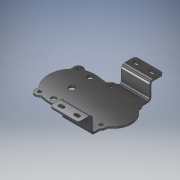
# Autodesk Inventor part: STEEL SIDE REDUCTION FRONT PLATE
Saved by Autodesk Inventor 2017 (Build 210142000, 142)
## iProperties
Part Number: STEEL SIDE REDUCTION FRONT PLATE
Material: Genérico
Document SubType Name: Modeling
Designer: Cristian
Density: 1 g/cm^3
Appearance: Valor por defecto
Author: Cristian
Autodesk Inventor part; units mm, degrees
ref_plane "XZ Plane" through (0, 0, 0) normal (0, 1, 0) x (-1, 0, 0)
ref_plane "XY Plane" through (0, 0, 0) normal (0, 0, 1) x (1, 0, 0)
sketch "Boceto1" plane through (0, 0, 0) normal (0, 0, 1) x (1, 0, 0)
  circle A0 centre (0, 0) radius 57.15
  circle A1 centre (101.6, 0) radius 44.45
  circle A2 centre (-31.75, 47.519) radius 11.1125
  circle A3 centre (-31.75, -47.519) radius 11.1125
  circle A4 centre (114.3, 42.5971) radius 11.1125
  circle A5 centre (114.3, -42.5971) radius 11.1125
  line L0 (7.1437, 56.7018) -> (107.1562, 44.1014)
  circle A6 centre (44.45, 52.0016) radius 11.1125
  line L1 (7.1437, -56.7018) -> (107.1562, -44.1014)
  circle A7 centre (44.45, -52.0016) radius 11.1125
  dimension "d0" = 114.3
  dimension "d1" = 88.9
  dimension "d2" = 203.2
  dimension "d3" = 22.225
  dimension "d4" = 22.225
  dimension "d7" = 22.225
  dimension "d8" = 22.225
  dimension "d11" = 22.225
  dimension "d13" = 0
  dimension "d14" = 22.225
  dimension "d35" = 31.75
  dimension "d36" = 31.75
  dimension "d37" = 44.45
  dimension "d38" = 44.45
  dimension "d39" = 12.7
  dimension "d40" = 12.7
  constraints: 8 centre point, 8 point on circle, 4 end point, 4 tangent, 2 point on line, 1 coincident
  measures "d0" diameter of A0
  measures "d1" diameter of A1
  measures "d3" diameter of A2
  measures "d4" diameter of A3
  measures "d7" diameter of A4
  measures "d8" diameter of A5
  measures "d11" diameter of A6
  measures "d13" vertical distance of point (0, 0) A1.centre
  measures "d14" diameter of A7
  measures "d35" horizontal distance of A0.centre A3.centre
  measures "d36" horizontal distance of A0.centre A2.centre
  measures "d37" horizontal distance of point (0, 0) A7.centre
  measures "d38" horizontal distance of point (0, 0) A6.centre
  measures "d39" horizontal distance of A1.centre A5.centre
  measures "d40" horizontal distance of A1.centre A4.centre
extrude "Extrusión1" add sketch "Boceto1" along normal blind 4.445
ref_plane "Plano de trabajo1" through (50.8, 0, 0) normal (1, 0, 0) x (0, 1, 0)
sketch "Boceto3" plane through (50.8, 0, 0) normal (1, 0, 0) x (0, 1, 0)
  line L0 (0, 0) -> (0, 4.445)
  line L1 (-52.7651, 4.445) -> (-56.7018, 4.445) projected
  line L2 (0, 4.445) -> (69.85, 4.445)
  line L3 (69.85, 4.445) -> (69.85, 44.45)
  line L4 (69.85, 44.45) -> (104.775, 44.45)
  line L5 (104.775, 44.45) -> (104.775, 40.005)
  line L6 (104.775, 40.005) -> (74.295, 40.005)
  line L7 (74.295, 40.005) -> (74.295, 0)
  line L8 (74.295, 0) -> (0, 0)
  point P0 (37.2916, 4.445)
  point P1 (-37.2916, 4.445)
  dimension "d28" = 4.445
  dimension "d29" = 4.445
  dimension "d30" = 69.85
  dimension "d31" = 44.45
  dimension "d32" = 104.775
  constraints: 16 end point, 6 perpendicular, 1 horizontal, 1 point on line
  measures "d28" distance between parallel lines of L7 L3
  measures "d29" distance between parallel lines of L4 L6
  measures "d30" distance of L0.end L2.end
  measures "d31" distance between parallel lines of L4 L8
  measures "d32" distance between parallel lines of L0 L5
extrude "Extrusión3" add sketch "Boceto3" along normal blind 69.85
fillet "Empalme3" radius 4.445 2 edges at (85.725, 69.85, 4.445) (85.725, 74.295, 40.005)
fillet "Empalme4" radius 8.89 2 edges at (85.725, 69.85, 44.45) (85.725, 74.295, 0)
sketch "Boceto4" plane through (50.8, 104.775, 44.45) normal (0, 0, 1) x (1, 0, 0)
  circle A0 centre (12.7254, -12.7254) radius 4.191
  circle A1 centre (19.0246, -12.7254) radius 4.191
  circle A2 centre (57.1246, -12.7254) radius 4.191
  circle A3 centre (50.8254, -12.7254) radius 4.191
  line L0 (57.1246, -8.5344) -> (50.8254, -8.5344)
  line L1 (57.1246, -16.9164) -> (50.8254, -16.9164)
  line L2 (0, 0) -> (69.85, 0) projected
  line L3 (69.85, 0) -> (69.85, -26.035) projected
  line L4 (19.0246, -8.5344) -> (12.7254, -8.5344)
  line L5 (12.7254, -16.9164) -> (19.0246, -16.9164)
  line L6 (0, -26.035) -> (0, 0) projected
  point P0 (-50.8, -104.775)
  point P1 (6.35, 0)
  point P2 (63.5, 0)
  point P3 (69.85, -6.35)
  point P4 (0, -6.35)
  dimension "d44" = 8.382
  dimension "d45" = 8.382
  dimension "d46" = 14.6812
  dimension "d47" = 8.5344
  dimension "d48" = 12.7254
  dimension "d49" = 8.382
  dimension "d50" = 8.382
  dimension "d51" = 14.6812
  dimension "d52" = 8.5344
  dimension "d53" = 12.7254
  constraints: 8 end point, 8 point on circle, 7 tangent, 4 centre point, 1 parallel
  measures "d44" diameter of A2
  measures "d45" diameter of A3
  measures "d47" distance between parallel lines of L2 L0
  measures "d48" distance from line of L3 A2.centre
  measures "d49" diameter of A1
  measures "d50" diameter of A0
  measures "d52" distance between parallel lines of L2 L4
  measures "d53" distance from line of L6 A0.centre
extrude "Extrusión4" cut sketch "Boceto4" against normal up to surface (4.445 mm away)
fillet "Empalme5" radius 6.35 2 edges at (120.65, 104.775, 42.2275) (50.8, 104.775, 42.2275)
mirror "Simetría1" about plane through (0, 0, 0) normal (0, 1, 0) of "Extrusión3", "Empalme3", "Empalme4", "Extrusión4", "Empalme5"
sketch "Boceto2" plane through (0, 0, 4.445) normal (0, 0, 1) x (1, 0, 0)
  arc A0 (-21.9537, 52.7651) -> (-40.3458, 40.4764) centre (-31.75, 47.519) ccw projected
  circle A1 centre (-31.75, 47.519) radius 4.2164
  arc A2 (-40.3458, -40.4764) -> (-21.9537, -52.7651) centre (-31.75, -47.519) ccw projected
  circle A3 centre (-31.75, -47.519) radius 4.2164
  arc A4 (33.4247, -53.3907) -> (55.4753, -50.6125) centre (44.45, -52.0016) ccw projected
  circle A5 centre (44.45, -52.0016) radius 4.2164
  arc A6 (55.4753, 50.6125) -> (33.4247, 53.3907) centre (44.45, 52.0016) ccw projected
  circle A7 centre (44.45, 52.0016) radius 4.2164
  arc A8 (124.4689, 38.1158) -> (103.3657, 44.5789) centre (114.3, 42.5971) ccw projected
  circle A9 centre (114.3, 42.5971) radius 4.2164
  arc A10 (103.3657, -44.5789) -> (124.4689, -38.1158) centre (114.3, -42.5971) ccw projected
  circle A11 centre (114.3, -42.5971) radius 4.2164
  point P0 (0, 0)
  dimension "d18" = 8.4328
  dimension "d19" = 8.4328
  dimension "d20" = 8.4328
  dimension "d21" = 8.4328
  dimension "d22" = 8.4328
  dimension "d23" = 8.4328
  constraints: 6 centre point, 6 coincident
  measures "d18" diameter of A1
  measures "d19" diameter of A3
  measures "d20" diameter of A5
  measures "d21" diameter of A7
  measures "d22" diameter of A9
  measures "d23" diameter of A11
extrude "Extrusión2" cut sketch "Boceto2" against normal up to surface (4.445 mm away)
fillet "Empalme6" radius 6.35 12 edges at (124.4689, 38.1158, 2.2225) (120.65, 51.7166, 2.2225) (-40.3458, 40.4764, 2.2225) (-21.9537, 52.7651, 2.2225) (124.4689, -38.1158, 2.2225) (120.65, -51.7166, 2.2225) (-21.9537, -52.7651, 2.2225) (-40.3458, -40.4764, 2.2225) (33.4247, -53.3907, 2.2225) (50.8, -61.1211, 2.2225) (50.8, 61.1211, 2.2225) (33.4247, 53.3907, 2.2225)
sketch "Boceto5" plane through (0, 0, 4.445) normal (0, 0, 1) x (1, 0, 0)
  circle A0 centre (0, 0) radius 7.1437
  line L0 (0, 0) -> (0, 45)
  line L1 (0, 0) -> (0, -45)
  circle A1 centre (0, 45) radius 6
  circle A2 centre (0, -45) radius 6
  dimension "d58" = 14.2875
  dimension "d59" = 45
  dimension "d60" = 45
  dimension "d61" = 12
  dimension "d62" = 12
  constraints: 4 end point, 3 centre point, 3 coincident, 2 vertical
  measures "d58" diameter of A0
  measures "d59" distance of L0.start L0.end
  measures "d60" distance of L0.start L1.end
  measures "d61" diameter of A1
  measures "d62" diameter of A2
extrude "Extrusión5" cut sketch "Boceto5" against normal up to surface (4.445 mm away)
equation "\"d16\" = t"
equation "\"d28\" = t"
equation "\"d29\" = t"
equation "\"d18\" = Q"
equation "\"d19\" = Q"
equation "\"d20\" = Q"
equation "\"d21\" = Q"
equation "\"d22\" = Q"
equation "\"d23\" = Q"
equation "\"d58\" = DF"
equation "\"d59\" = 0.5 * JF"
equation "\"d60\" = 0.5 * JF"
equation "\"d61\" = NF"
equation "\"d62\" = NF"
equation "\"t\" = 4.445"
equation "\"Q\" = 8.4328"
equation "\"DF\" = 14.2875"
equation "\"NF\" = 12"
equation "\"JF\" = 90"
